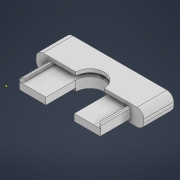
# Autodesk Inventor part: syringe_fitter
Saved by Autodesk Inventor 2022 (Build 260153000, 153)
## iProperties
Created: 2023-04-21
Part Number: syringe_fitter
Material: Generic
Document SubType Name: Modeling
Designer: Jakob Saugbjerg
Density: 1 g/cm^3
Appearance: Default
Author: Jakob Saugbjerg
Autodesk Inventor part; units mm, degrees
ref_plane "YZ Plane" through (0, 0, 0) normal (1, 0, 0) x (0, 1, 0)
ref_plane "XZ Plane" through (0, 0, 0) normal (0, 1, 0) x (-1, 0, 0)
ref_plane "XY Plane" through (0, 0, 0) normal (0, 0, 1) x (1, 0, 0)
sketch "Sketch13" plane through (0, 0, 0) normal (0, 0, 1) x (1, 0, 0)
  line L0 (0, 0) -> (63, 0)
  line L1 (63, 0) -> (63, 10)
  line L2 (63, 10) -> (0, 10)
  line L3 (0, 10) -> (0, 0)
  dimension "d38" = 63
  dimension "d39" = 10
  constraints: 8 end point, 2 parallel, 1 horizontal, 1 perpendicular
  measures "d38" distance of L2.end L1.end
  measures "d39" distance of L1.end L0.end
extrude "Extrusion8" add sketch "Sketch13" along normal blind 35
sketch "Sketch15" plane through (0, 10, 0) normal (0, 1, 0) x (1, 0, 0)
  line L0 (63, -35) -> (0, -35) projected
  line L1 (31.5, -35) -> (31.5, -17.5)
  circle A0 centre (31.5, -17.5) radius 8.25
  line L2 (44, -35) -> (23.25, -35)
  line L3 (23.25, -35) -> (23.25, -17.5)
  line L4 (39.75, -17.5) -> (39.75, -35)
  point P0 (0, 0)
  dimension "d42" = 17.5
  dimension "d43" = 16.5
  constraints: 8 end point, 2 point on circle, 2 point on line, 1 centre point, 1 coincident, 1 midpoint, 1 perpendicular, 1 vertical
  measures "d42" distance of L1.start L1.end
  measures "d43" diameter of A0
extrude "Extrusion9" cut sketch "Sketch15" against normal blind 35
sketch "Sketch16" plane through (0, 10, 0) normal (0, 1, 0) x (1, 0, 0)
  line L0 (0, -35) -> (23.25, -35) projected
  line L1 (0, -35) -> (63, -35)
  line L2 (63, -35) -> (63, -17.5)
  line L3 (63, -17.5) -> (0, -17.5)
  line L4 (0, -17.5) -> (0, -35)
  point P0 (0, 0)
  dimension "d46" = 63
  dimension "d47" = 17.5
  constraints: 8 end point, 2 parallel, 1 horizontal, 1 perpendicular
  measures "d46" distance of L3.end L2.end
  measures "d47" distance of L2.end L1.end
extrude "Extrusion10" cut sketch "Sketch16" against normal blind 2
sketch "Sketch17" plane through (0, 0, 0) normal (0, -1, 0) x (1, 0, 0)
  line L0 (0, 35) -> (23.25, 35) projected
  line L1 (63, 0) -> (63, 35) projected
  line L2 (0, 35) -> (63, 35)
  line L3 (63, 35) -> (63, 17.5)
  line L4 (63, 17.5) -> (0, 17.5)
  line L5 (0, 17.5) -> (0, 35)
  dimension "d70" = 17.5
  constraints: 8 end point, 2 parallel, 1 horizontal, 1 midpoint, 1 perpendicular
  measures "d70" distance of L2.end L3.end
extrude "Extrusion11" cut sketch "Sketch17" against normal blind 2
sketch "Sketch19" plane through (0, 0, 35) normal (0, 0, 1) x (1, 0, 0)
  line L0 (23.25, 8) -> (0, 8) projected
  line L1 (9.5, 8) -> (53.5, 8)
  line L2 (53.5, 8) -> (53.5, 6)
  line L3 (53.5, 6) -> (9.5, 6)
  line L4 (9.5, 6) -> (9.5, 8)
  point P0 (0, 0)
  dimension "d68" = 2
  constraints: 8 end point, 2 parallel, 1 horizontal, 1 perpendicular, 1 point on line
  measures "d68" distance of L1.end L2.end
extrude "Extrusion12" cut sketch "Sketch19" against normal blind 33
fillet "Fillet5" radius 2 2 edges at (9.5, 7, 35) (53.5, 7, 35)
sketch "Sketch20" plane through (0, 0, 35) normal (0, 0, 1) x (1, 0, 0)
  line L0 (63, 8) -> (39.75, 8) projected
  line L1 (7.5, 2) -> (55.5, 2)
  line L2 (55.5, 2) -> (55.5, 8)
  line L3 (55.5, 8) -> (7.5, 8)
  line L4 (7.5, 8) -> (7.5, 2)
  line L5 (7.5, 2) -> (55.5, 8) construction
  line L6 (55.5, 2) -> (7.5, 8) construction
  line L7 (7.5, 8) -> (0, 8)
  line L8 (0, 8) -> (0, 2)
  line L9 (0, 2) -> (7.5, 2)
  line L10 (7.5, 2) -> (7.5, 8)
  line L11 (39.75, 2) -> (63, 2) projected
  line L12 (55.5, 8) -> (63, 8)
  line L13 (63, 8) -> (63, 2)
  line L14 (63, 2) -> (55.5, 2)
  line L15 (55.5, 2) -> (55.5, 8)
  point P0 (0, 0)
  point P1 (31.5, 5)
  point P2 (55.5, 2)
  dimension "d58" = 48
  constraints: 28 end point, 6 parallel, 3 horizontal, 3 perpendicular, 2 midpoint, 1 point on line
  measures "d58" distance of L3.end L2.end
extrude "Extrusion13" cut sketch "Sketch20" against normal blind 17.5 contours L13 L11 L2 L0 | L4 L9 L8 L7
fillet "Fillet6" radius 1 4 edges at (55.5, 2, 26.25) (55.5, 8, 26.25) (7.5, 8, 26.25) (7.5, 2, 26.25)
sketch "Sketch21" plane through (0, 0, 0) normal (0, 0, -1) x (-1, 0, 0)
  line L0 (-42.4052, 3.635) -> (-43.8922, 3.635)
  line L1 (-43.8922, 3.635) -> (-43.8922, 3.9462)
  line L2 (-43.8922, 3.9462) -> (-43.3389, 3.9462)
  line L3 (-43.3389, 3.9462) -> (-43.3389, 5.9889)
  line L4 (-43.3389, 5.9889) -> (-43.8922, 5.9889)
  line L5 (-43.8922, 5.9889) -> (-43.8922, 6.268)
  spline S0 degree 2 poles (-43.8922, 6.268) (-43.5785, 6.268) (-43.2821, 6.4459) (-43.2623, 6.6929) knots 0 0 0 1 2 2 2
  line L6 (-43.2623, 6.6929) -> (-42.9462, 6.6929)
  line L7 (-42.9462, 6.6929) -> (-42.9462, 3.9462)
  line L8 (-42.9462, 3.9462) -> (-42.4052, 3.9462)
  line L9 (-42.4052, 3.9462) -> (-42.4052, 3.635)
  spline S1 degree 2 poles (-39.9476, 5.159) (-39.9476, 4.339) (-40.4243, 3.5708) (-40.9208, 3.5708) knots 0 0 0 1 2 2 2
  spline S2 degree 2 poles (-40.9208, 3.5708) (-41.4246, 3.5708) (-41.8964, 4.3538) (-41.8964, 5.1565) knots 0 0 0 1 2 2 2
  spline S3 degree 2 poles (-41.8964, 5.1565) (-41.8964, 5.9815) (-41.4197, 6.7448) (-40.9208, 6.7448) knots 0 0 0 1 2 2 2
  spline S4 degree 2 poles (-40.9208, 6.7448) (-40.4194, 6.7448) (-39.9476, 5.9543) (-39.9476, 5.159) knots 0 0 0 1 2 2 2
  spline S5 degree 2 poles (-40.4712, 4.2303) (-40.4119, 4.3809) (-40.3625, 4.8453) (-40.3625, 5.159) knots 0 0 0 1 2 2 2
  spline S6 degree 2 poles (-40.3625, 5.159) (-40.3625, 5.4727) (-40.4119, 5.9346) (-40.4737, 6.0902) knots 0 0 0 1 2 2 2
  spline S7 degree 2 poles (-40.4737, 6.0902) (-40.5354, 6.2458) (-40.7503, 6.4064) (-40.9208, 6.4064) knots 0 0 0 1 2 2 2
  spline S8 degree 2 poles (-40.9208, 6.4064) (-41.0912, 6.4064) (-41.311, 6.2458) (-41.3752, 6.0853) knots 0 0 0 1 2 2 2
  spline S9 degree 2 poles (-41.3752, 6.0853) (-41.437, 5.9296) (-41.4815, 5.4554) (-41.4815, 5.1565) knots 0 0 0 1 2 2 2
  spline S10 degree 2 poles (-41.4815, 5.1565) (-41.4815, 4.8354) (-41.4419, 4.4056) (-41.3777, 4.2377) knots 0 0 0 1 2 2 2
  spline S11 degree 2 poles (-41.3777, 4.2377) (-41.3184, 4.0796) (-41.0986, 3.9092) (-40.9208, 3.9092) knots 0 0 0 1 2 2 2
  spline S12 degree 2 poles (-40.9208, 3.9092) (-40.7528, 3.9092) (-40.533, 4.0697) (-40.4712, 4.2303) knots 0 0 0 1 2 2 2
  line L10 (-35.5979, 3.635) -> (-35.5979, 4.9589)
  spline S13 degree 2 poles (-35.5979, 4.9589) (-35.5979, 5.117) (-35.6226, 5.3862) (-35.6621, 5.4603) knots 0 0 0 1 2 2 2
  spline S14 degree 2 poles (-35.6621, 5.4603) (-35.7016, 5.5419) (-35.8523, 5.6209) (-35.9832, 5.6209) knots 0 0 0 1 2 2 2
  spline S15 degree 2 poles (-35.9832, 5.6209) (-36.1018, 5.6209) (-36.3735, 5.4752) (-36.5167, 5.3368) knots 0 0 0 1 2 2 2
  spline S16 degree 2 poles (-36.5167, 5.3368) (-36.5143, 5.3023) (-36.5093, 5.2059) (-36.5093, 5.1417) knots 0 0 0 1 2 2 2
  line L11 (-36.5093, 5.1417) -> (-36.5093, 3.635)
  line L12 (-36.5093, 3.635) -> (-36.8946, 3.635)
  line L13 (-36.8946, 3.635) -> (-36.8946, 4.9589)
  spline S17 degree 2 poles (-36.8946, 4.9589) (-36.8946, 5.117) (-36.9193, 5.3862) (-36.9589, 5.4603) knots 0 0 0 1 2 2 2
  spline S18 degree 2 poles (-36.9589, 5.4603) (-36.9984, 5.5419) (-37.1491, 5.6209) (-37.28, 5.6209) knots 0 0 0 1 2 2 2
  spline S19 degree 2 poles (-37.28, 5.6209) (-37.4035, 5.6209) (-37.6776, 5.4653) (-37.8061, 5.3443) knots 0 0 0 1 2 2 2
  line L14 (-37.8061, 5.3443) -> (-37.8061, 3.635)
  line L15 (-37.8061, 3.635) -> (-38.1914, 3.635)
  line L16 (-38.1914, 3.635) -> (-38.1914, 5.9222)
  line L17 (-38.1914, 5.9222) -> (-37.8061, 5.9222)
  line L18 (-37.8061, 5.9222) -> (-37.8061, 5.6703)
  spline S20 degree 2 poles (-37.8061, 5.6703) (-37.6554, 5.821) (-37.359, 5.9865) (-37.1812, 5.9865) knots 0 0 0 1 2 2 2
  spline S21 degree 2 poles (-37.1812, 5.9865) (-36.9786, 5.9865) (-36.6649, 5.8012) (-36.5834, 5.5913) knots 0 0 0 1 2 2 2
  spline S22 degree 2 poles (-36.5834, 5.5913) (-36.408, 5.7864) (-36.0771, 5.9865) (-35.8844, 5.9865) knots 0 0 0 1 2 2 2
  spline S23 degree 2 poles (-35.8844, 5.9865) (-35.7362, 5.9865) (-35.4941, 5.8951) (-35.4052, 5.7913) knots 0 0 0 1 2 2 2
  spline S24 degree 2 poles (-35.4052, 5.7913) (-35.3138, 5.6876) (-35.2126, 5.3764) (-35.2126, 5.1417) knots 0 0 0 1 2 2 2
  line L19 (-35.2126, 5.1417) -> (-35.2126, 3.635)
  line L20 (-35.2126, 3.635) -> (-35.5979, 3.635)
  line L21 (-32.8759, 3.635) -> (-34.642, 3.635)
  line L22 (-34.642, 3.635) -> (-34.642, 6.683)
  line L23 (-34.642, 6.683) -> (-34.2369, 6.683)
  line L24 (-34.2369, 6.683) -> (-34.2369, 3.9956)
  line L25 (-34.2369, 3.9956) -> (-32.8759, 3.9956)
  line L26 (-32.8759, 3.9956) -> (-32.8759, 3.635)
  spline S25 degree 2 poles (-30.6603, 3.5807) (-30.89, 3.5807) (-31.2877, 3.7042) (-31.4186, 3.7733) knots 0 0 0 1 2 2 2
  line L27 (-31.4186, 3.7733) -> (-31.4186, 4.2056)
  line L28 (-31.4186, 4.2056) -> (-31.3989, 4.2056)
  spline S26 degree 2 poles (-31.3989, 4.2056) (-31.3495, 4.1661) (-31.2161, 4.0722) (-31.1049, 4.0203) knots 0 0 0 1 2 2 2
  spline S27 degree 2 poles (-31.1049, 4.0203) (-31.0086, 3.9734) (-30.7715, 3.9042) (-30.6455, 3.9042) knots 0 0 0 1 2 2 2
  spline S28 degree 2 poles (-30.6455, 3.9042) (-30.5541, 3.9042) (-30.3442, 3.9462) (-30.2948, 3.9808) knots 0 0 0 1 2 2 2
  spline S29 degree 2 poles (-30.2948, 3.9808) (-30.2231, 4.0277) (-30.1589, 4.1339) (-30.1589, 4.2426) knots 0 0 0 1 2 2 2
  spline S30 degree 2 poles (-30.1589, 4.2426) (-30.1589, 4.3785) (-30.3071, 4.5193) (-30.4973, 4.5662) knots 0 0 0 1 2 2 2
  spline S31 degree 2 poles (-30.4973, 4.5662) (-30.5714, 4.5835) (-30.8085, 4.6329) (-30.9098, 4.6601) knots 0 0 0 1 2 2 2
  spline S32 degree 2 poles (-30.9098, 4.6601) (-31.1716, 4.7366) (-31.4087, 5.0528) (-31.4087, 5.2776) knots 0 0 0 1 2 2 2
  spline S33 degree 2 poles (-31.4087, 5.2776) (-31.4087, 5.5888) (-30.9419, 5.9766) (-30.5566, 5.9766) knots 0 0 0 1 2 2 2
  spline S34 degree 2 poles (-30.5566, 5.9766) (-30.3664, 5.9766) (-29.9811, 5.8827) (-29.8502, 5.8111) knots 0 0 0 1 2 2 2
  line L29 (-29.8502, 5.8111) -> (-29.8502, 5.3986)
  line L30 (-29.8502, 5.3986) -> (-29.8699, 5.3986)
  spline S35 degree 2 poles (-29.8699, 5.3986) (-30.0181, 5.5172) (-30.3787, 5.653) (-30.564, 5.653) knots 0 0 0 1 2 2 2
  spline S36 degree 2 poles (-30.564, 5.653) (-30.7542, 5.653) (-31.016, 5.4925) (-31.016, 5.3319) knots 0 0 0 1 2 2 2
  spline S37 degree 2 poles (-31.016, 5.3319) (-31.016, 5.1862) (-30.8604, 5.0454) (-30.6875, 5.0009) knots 0 0 0 1 2 2 2
  spline S38 degree 2 poles (-30.6875, 5.0009) (-30.6035, 4.9787) (-30.3911, 4.9342) (-30.275, 4.9071) knots 0 0 0 1 2 2 2
  spline S39 degree 2 poles (-30.275, 4.9071) (-30.0231, 4.8428) (-29.7662, 4.5489) (-29.7662, 4.2945) knots 0 0 0 1 2 2 2
  spline S40 degree 2 poles (-29.7662, 4.2945) (-29.7662, 4.1463) (-29.8823, 3.8845) (-29.9959, 3.7881) knots 0 0 0 1 2 2 2
  spline S41 degree 2 poles (-29.9959, 3.7881) (-30.1169, 3.6869) (-30.4257, 3.5807) (-30.6603, 3.5807) knots 0 0 0 1 2 2 2
  line L31 (-27.6123, 5.9222) -> (-28.8424, 2.7927)
  line L32 (-28.8424, 2.7927) -> (-29.2549, 2.7927)
  line L33 (-29.2549, 2.7927) -> (-28.8449, 3.7462)
  line L34 (-28.8449, 3.7462) -> (-29.6748, 5.9222)
  line L35 (-29.6748, 5.9222) -> (-29.2598, 5.9222)
  line L36 (-29.2598, 5.9222) -> (-28.6349, 4.2278)
  line L37 (-28.6349, 4.2278) -> (-28.0125, 5.9222)
  line L38 (-28.0125, 5.9222) -> (-27.6123, 5.9222)
  line L39 (-26.1081, 5.5097) -> (-26.1278, 5.5097)
  spline S42 degree 2 poles (-26.1278, 5.5097) (-26.1723, 5.5221) (-26.2686, 5.527) (-26.3353, 5.527) knots 0 0 0 1 2 2 2
  spline S43 degree 2 poles (-26.3353, 5.527) (-26.4909, 5.527) (-26.7972, 5.3912) (-26.9355, 5.2578) knots 0 0 0 1 2 2 2
  line L40 (-26.9355, 5.2578) -> (-26.9355, 3.635)
  line L41 (-26.9355, 3.635) -> (-27.3209, 3.635)
  line L42 (-27.3209, 3.635) -> (-27.3209, 5.9222)
  line L43 (-27.3209, 5.9222) -> (-26.9355, 5.9222)
  line L44 (-26.9355, 5.9222) -> (-26.9355, 5.5814)
  spline S44 degree 2 poles (-26.9355, 5.5814) (-26.7256, 5.7691) (-26.4119, 5.9222) (-26.2637, 5.9222) knots 0 0 0 1 2 2 2
  spline S45 degree 2 poles (-26.2637, 5.9222) (-26.2044, 5.9222) (-26.1451, 5.9173) (-26.1081, 5.9099) knots 0 0 0 1 2 2 2
  line L45 (-26.1081, 5.9099) -> (-26.1081, 5.5097)
  line L46 (-25.4165, 3.635) -> (-25.8018, 3.635)
  line L47 (-25.8018, 3.635) -> (-25.8018, 5.9222)
  line L48 (-25.8018, 5.9222) -> (-25.4165, 5.9222)
  line L49 (-25.4165, 5.9222) -> (-25.4165, 3.635)
  line L50 (-25.3893, 6.3026) -> (-25.8265, 6.3026)
  line L51 (-25.8265, 6.3026) -> (-25.8265, 6.7028)
  line L52 (-25.8265, 6.7028) -> (-25.3893, 6.7028)
  line L53 (-25.3893, 6.7028) -> (-25.3893, 6.3026)
  line L54 (-23.0551, 3.635) -> (-23.4405, 3.635)
  line L55 (-23.4405, 3.635) -> (-23.4405, 4.9392)
  spline S46 degree 2 poles (-23.4405, 4.9392) (-23.4405, 5.0973) (-23.4701, 5.369) (-23.5146, 5.4505) knots 0 0 0 1 2 2 2
  spline S47 degree 2 poles (-23.5146, 5.4505) (-23.5615, 5.5369) (-23.7295, 5.6209) (-23.8727, 5.6209) knots 0 0 0 1 2 2 2
  spline S48 degree 2 poles (-23.8727, 5.6209) (-24.016, 5.6209) (-24.3198, 5.4678) (-24.4655, 5.3443) knots 0 0 0 1 2 2 2
  line L56 (-24.4655, 5.3443) -> (-24.4655, 3.635)
  line L57 (-24.4655, 3.635) -> (-24.8508, 3.635)
  line L58 (-24.8508, 3.635) -> (-24.8508, 5.9222)
  line L59 (-24.8508, 5.9222) -> (-24.4655, 5.9222)
  line L60 (-24.4655, 5.9222) -> (-24.4655, 5.6678)
  spline S49 degree 2 poles (-24.4655, 5.6678) (-24.2926, 5.8234) (-23.9592, 5.9865) (-23.7714, 5.9865) knots 0 0 0 1 2 2 2
  spline S50 degree 2 poles (-23.7714, 5.9865) (-23.4355, 5.9865) (-23.0551, 5.5419) (-23.0551, 5.1195) knots 0 0 0 1 2 2 2
  line L61 (-23.0551, 5.1195) -> (-23.0551, 3.635)
  spline S51 degree 2 poles (-22.4327, 3.2694) (-22.3932, 3.2522) (-22.2425, 3.1978) (-22.1462, 3.1756) knots 0 0 0 1 2 2 2
  spline S52 degree 2 poles (-22.1462, 3.1756) (-22.04, 3.1484) (-21.8596, 3.1163) (-21.7534, 3.1163) knots 0 0 0 1 2 2 2
  spline S53 degree 2 poles (-21.7534, 3.1163) (-21.5756, 3.1163) (-21.3286, 3.2102) (-21.2594, 3.2941) knots 0 0 0 1 2 2 2
  spline S54 degree 2 poles (-21.2594, 3.2941) (-21.1927, 3.3781) (-21.1409, 3.598) (-21.1409, 3.7387) knots 0 0 0 1 2 2 2
  line L62 (-21.1409, 3.7387) -> (-21.1409, 3.9388)
  spline S55 degree 2 poles (-21.1409, 3.9388) (-21.2965, 3.803) (-21.5954, 3.6745) (-21.8201, 3.6745) knots 0 0 0 1 2 2 2
  spline S56 degree 2 poles (-21.8201, 3.6745) (-22.2104, 3.6745) (-22.6723, 4.255) (-22.6723, 4.8009) knots 0 0 0 1 2 2 2
  spline S57 degree 2 poles (-22.6723, 4.8009) (-22.6723, 5.0849) (-22.5117, 5.5246) (-22.3784, 5.6802) knots 0 0 0 1 2 2 2
  spline S58 degree 2 poles (-22.3784, 5.6802) (-22.2499, 5.8259) (-21.8967, 5.9865) (-21.709, 5.9865) knots 0 0 0 1 2 2 2
  spline S59 degree 2 poles (-21.709, 5.9865) (-21.5311, 5.9865) (-21.2718, 5.9025) (-21.1409, 5.8259) knots 0 0 0 1 2 2 2
  line L63 (-21.1409, 5.8259) -> (-21.1186, 5.9222)
  line L64 (-21.1186, 5.9222) -> (-20.7556, 5.9222)
  line L65 (-20.7556, 5.9222) -> (-20.7556, 3.8968)
  spline S60 degree 2 poles (-20.7556, 3.8968) (-20.7556, 3.3139) (-21.2619, 2.7705) (-21.7831, 2.7705) knots 0 0 0 1 2 2 2
  spline S61 degree 2 poles (-21.7831, 2.7705) (-21.951, 2.7705) (-22.3018, 2.8248) (-22.4525, 2.8693) knots 0 0 0 1 2 2 2
  line L66 (-22.4525, 2.8693) -> (-22.4525, 3.2694)
  line L67 (-22.4525, 3.2694) -> (-22.4327, 3.2694)
  line L68 (-21.1409, 4.255) -> (-21.1409, 5.5122)
  spline S62 degree 2 poles (-21.1409, 5.5122) (-21.2841, 5.5814) (-21.5262, 5.6407) (-21.6472, 5.6407) knots 0 0 0 1 2 2 2
  spline S63 degree 2 poles (-21.6472, 5.6407) (-21.9387, 5.6407) (-22.2746, 5.2109) (-22.2746, 4.8083) knots 0 0 0 1 2 2 2
  spline S64 degree 2 poles (-22.2746, 4.8083) (-22.2746, 4.4279) (-22.0202, 4.0302) (-21.7337, 4.0302) knots 0 0 0 1 2 2 2
  spline S65 degree 2 poles (-21.7337, 4.0302) (-21.583, 4.0302) (-21.2668, 4.1488) (-21.1409, 4.255) knots 0 0 0 1 2 2 2
  spline S66 degree 2 poles (-19.2044, 3.5831) (-19.7527, 3.5831) (-20.3554, 4.1982) (-20.3554, 4.7663) knots 0 0 0 1 2 2 2
  spline S67 degree 2 poles (-20.3554, 4.7663) (-20.3554, 5.3245) (-19.77, 5.9865) (-19.2982, 5.9865) knots 0 0 0 1 2 2 2
  spline S68 degree 2 poles (-19.2982, 5.9865) (-19.0858, 5.9865) (-18.7573, 5.863) (-18.6363, 5.732) knots 0 0 0 1 2 2 2
  spline S69 degree 2 poles (-18.6363, 5.732) (-18.5128, 5.6011) (-18.3819, 5.2232) (-18.3819, 4.9491) knots 0 0 0 1 2 2 2
  line L69 (-18.3819, 4.9491) -> (-18.3819, 4.7391)
  line L70 (-18.3819, 4.7391) -> (-19.9651, 4.7391)
  spline S70 degree 2 poles (-19.9651, 4.7391) (-19.9651, 4.3414) (-19.565, 3.9191) (-19.2093, 3.9191) knots 0 0 0 1 2 2 2
  spline S71 degree 2 poles (-19.2093, 3.9191) (-19.0834, 3.9191) (-18.8388, 3.9759) (-18.74, 4.0203) knots 0 0 0 1 2 2 2
  spline S72 degree 2 poles (-18.74, 4.0203) (-18.6363, 4.0697) (-18.493, 4.1562) (-18.4461, 4.1957) knots 0 0 0 1 2 2 2
  line L71 (-18.4461, 4.1957) -> (-18.4239, 4.1957)
  line L72 (-18.4239, 4.1957) -> (-18.4239, 3.7758)
  spline S73 degree 2 poles (-18.4239, 3.7758) (-18.4905, 3.7486) (-18.6931, 3.6696) (-18.7721, 3.6474) knots 0 0 0 1 2 2 2
  spline S74 degree 2 poles (-18.7721, 3.6474) (-18.8833, 3.6152) (-19.0661, 3.5831) (-19.2044, 3.5831) knots 0 0 0 1 2 2 2
  spline S75 degree 2 poles (-18.7573, 5.033) (-18.7622, 5.1886) (-18.8265, 5.4159) (-18.8882, 5.4925) knots 0 0 0 1 2 2 2
  spline S76 degree 2 poles (-18.8882, 5.4925) (-18.9549, 5.5789) (-19.1649, 5.6703) (-19.3205, 5.6703) knots 0 0 0 1 2 2 2
  spline S77 degree 2 poles (-19.3205, 5.6703) (-19.4736, 5.6703) (-19.6885, 5.5789) (-19.7774, 5.49) knots 0 0 0 1 2 2 2
  spline S78 degree 2 poles (-19.7774, 5.49) (-19.8639, 5.3986) (-19.9528, 5.1788) (-19.9651, 5.033) knots 0 0 0 1 2 2 2
  line L73 (-19.9651, 5.033) -> (-18.7573, 5.033)
  point P0 (0, 0)
  point P1 (-44.3541, 6.7448)
  dimension "d39" = 10
  constraints: 1 other
emboss "Emboss3" sketch "Sketch21" operation cut depth 1 direction (0, 0, 1)
sketch "Sketch22" plane through (0, 0, 35) normal (0, 0, 1) x (1, 0, 0)
  point P0 (0, 0)
sketch "Sketch23" plane through (55.5, 3, 17.5) normal (1, 0, 0) x (0, 0, -1)
  line L0 (-15.5, 5) -> (0, 5) projected
  line L1 (-17.5, -1) -> (-17.5, 0) projected
  line L2 (0, 5) -> (-17.5, 5)
  line L3 (-17.5, 5) -> (-17.5, -1)
  line L4 (-17.5, -1) -> (0, -1)
  line L5 (0, -1) -> (0, 5)
  point P0 (17.5, -3)
  constraints: 8 end point, 2 parallel, 1 horizontal, 1 perpendicular
extrude "Extrusion14" cut sketch "Sketch23" against normal blind 0.2
sketch "Sketch24" plane through (7.5, 3, 17.5) normal (-1, 0, 0) x (0, 0, 1)
  line L0 (0, 5) -> (15.5, 5) projected
  line L1 (0, -1) -> (17.5, -1) projected
  line L2 (0, 5) -> (17.5, 5)
  line L3 (17.5, 5) -> (17.5, -1)
  line L4 (17.5, -1) -> (0, -1)
  line L5 (0, -1) -> (0, 5)
  point P0 (-17.5, -3)
  point P1 (2.5, -1)
  point P2 (2.5, -1)
  constraints: 8 end point, 2 parallel, 1 horizontal, 1 perpendicular
extrude "Extrusion15" cut sketch "Sketch24" against normal blind 0.2
fillet "Fillet7" radius 4 4 edges at (0, 10, 8.75) (0, 0, 8.75) (63, 10, 8.75) (63, 0, 8.75)
sketch "Sketch25" plane through (0, 0, 35) normal (0, 0, 1) x (1, 0, 0)
  point P0 (0, 0)
body "Solid2"
